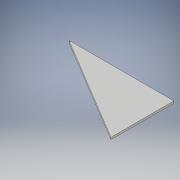
# Autodesk Inventor part: bottom-playfield
Saved by Autodesk Inventor 2017 (Build 210142000, 142)
## iProperties
Created: 2017-03-02
Part Number: bottom-playfield
Material: Generic
Document SubType Name: Modeling
Designer: John
Density: 1 g/cm^3
Appearance: Default
Author: John
Autodesk Inventor part; units mm, degrees
ref_plane "YZ Plane" through (0, 0, 0) normal (1, 0, 0) x (0, 1, 0)
ref_plane "XZ Plane" through (0, 0, 0) normal (0, 1, 0) x (-1, 0, 0)
ref_plane "XY Plane" through (0, 0, 0) normal (0, 0, 1) x (1, 0, 0)
sketch "Sketch1" plane through (0, 0, 0) normal (0, 1, 0) x (-1, 0, 0)
  line L0 (150, 0) -> (0, 90) construction
  line L1 (0, 90) -> (0, 0)
  line L2 (0, 0) -> (150, 0)
  line L3 (0, 90) -> (150, 0)
  point P0 (0, 0)
  dimension "d5" = 0
  dimension "d8" = 150
  dimension "d9" = 90
  constraints: 8 end point, 1 perpendicular, 1 vertical
  measures "d5" distance of L1.end point (0, 0)
  measures "d8" distance of L1.end L0.start
  measures "d9" distance of L0.end L1.end
extrude "Extrusion1" add sketch "Sketch1" along normal blind 3
body "Solid1"
